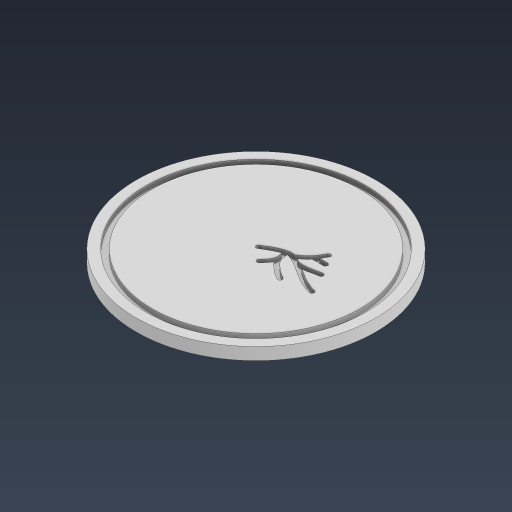
# Autodesk Inventor part: Podkladka_serce
Saved by Autodesk Inventor 2024 (Build 280153000, 153)
## iProperties
Created: 2023-12-26
Part Number: Podkladka_serce
Material: Generic
Document SubType Name: Modeling
Designer: Piter
Density: 1 g/cm^3
Appearance: Default
Author: Piter
Autodesk Inventor part; units mm, degrees
ref_plane "YZ Plane" through (0, 0, 0) normal (1, 0, 0) x (0, 1, 0)
ref_plane "XZ Plane" through (0, 0, 0) normal (0, 1, 0) x (-1, 0, 0)
ref_plane "XY Plane" through (0, 0, 0) normal (0, 0, 1) x (1, 0, 0)
sketch "Sketch1" plane through (0, 0, 0) normal (0, 1, 0) x (-1, 0, 0)
  circle A0 centre (0, 0) radius 49
  dimension "d0" = 98
  constraints: 1 centre point, 1 coincident
  measures "d0" diameter of A0
extrude "Extrusion1" add sketch "Sketch1" along normal blind 5
sketch "Sketch2" plane through (0, 5, 0) normal (0, 1, 0) x (1, 0, 0)
  circle A0 centre (0, 0) radius 45
  circle A1 centre (0, 0) radius 42.5
  dimension "d3" = 90
  dimension "d4" = 85
  constraints: 2 centre point, 2 coincident
  measures "d3" diameter of A0
  measures "d4" diameter of A1
extrude "Extrusion2" cut sketch "Sketch2" against normal blind 2
sketch "Sketch3" plane through (0, 5, 0) normal (0, 1, 0) x (1, 0, 0)
  line L0 (-57.9545, -56.5544) -> (-57.9545, 60.4671) construction
  line L1 (-57.9545, 60.4671) -> (59.0671, 60.4671) construction
  line L2 (59.0671, 60.4671) -> (59.0671, -56.5544) construction
  line L3 (59.0671, -56.5544) -> (-57.9545, -56.5544) construction
  spline S0 degree 4 poles (-30.855, -14.6939) (-30.5592, -15.2121) (-28.9514, -13.3397) (-26.9762, -13.2223) (-24.8329, -11.8951) (-22.2326, -11.9313) (-20.944, -12.0116) (-19.8559, -12.2221) (-18.785, -12.2474) (-17.611, -12.515) (-16.3643, -12.7351) (-15.334, -13.394) (-15.132, -13.7512) knots 0 0 0 0 0 0.211335 0.31885 0.420472 0.514533 0.599869 0.673378 0.744824 0.818641 1 1 1 1 1
  spline S1 degree 4 poles (-15.132, -13.7512) (-14.8227, -14.055) (-14.7175, -14.4119) (-14.2396, -15.0741) (-13.9799, -15.4717) (-13.6078, -15.8281) (-13.4414, -16.0861) (-13.1181, -16.4937) (-12.8312, -16.729) (-12.5324, -17.1008) (-12.243, -17.2913) (-11.898, -17.6305) (-11.433, -17.931) (-11.1614, -18.1872) (-10.7354, -18.4386) (-10.393, -18.6914) (-10.1007, -18.8902) (-9.6444, -19.1399) (-9.4269, -19.2823) (-8.8905, -19.4957) (-8.5475, -19.6618) (-8.2328, -19.8231) (-8.0583, -19.8821) knots 0 0 0 0 0 0.130277 0.178357 0.223468 0.267757 0.312685 0.357477 0.402319 0.447217 0.493758 0.540064 0.587831 0.634826 0.679831 0.725599 0.769028 0.811962 0.854881 0.896603 1 1 1 1 1
  spline S2 degree 4 poles (-8.0583, -19.8821) (-7.8236, -19.9246) (-7.3928, -20.2345) (-7.0213, -20.2224) (-6.4723, -20.5412) (-5.7818, -20.6348) (-4.0839, -21.2438) (-2.8883, -21.2479) (-2.0598, -21.5949) (3.0382, -21.8666) (4.3318, -21.5299) (5.1217, -21.4873) knots 0 0 0 0 0 0.143312 0.201694 0.275908 0.361306 0.452284 0.563274 0.684961 1 1 1 1 1
  spline S3 degree 4 poles (5.1217, -21.4873) (5.3502, -21.885) (7.9688, -22.2735) (9.7694, -21.9854) (13.5046, -20.8683) (15.0412, -20.3002) (18.2153, -18.4381) (18.9378, -17.9974) (21.8671, -15.9314) (23.6336, -14.3654) (24.9433, -13.2213) (28.1026, -10.9236) (30.8845, -9.4621) (34.5176, -7.4895) (35.0528, -6.595) (36.3359, -4.3458) knots 0 0 0 0 0 0.142124 0.208489 0.276802 0.341864 0.408085 0.475147 0.538695 0.609209 0.678841 0.750076 0.822266 1 1 1 1 1
  spline S4 degree 4 poles (36.3359, -4.3458) (36.7245, -3.6239) (36.8383, -0.8543) (35.4768, 2.2728) (32.0422, 7.8368) (27.8466, 12.0021) (23.4613, 16.0926) (18.9758, 17.9098) (17.0368, 19.1716) (10.9838, 20.2095) (4.2523, 20.1992) (2.4357, 19.9615) (-5.0655, 18.757) (-6.5918, 17.9988) knots 0 0 0 0 0 0.146469 0.225498 0.31307 0.401766 0.484157 0.564599 0.642138 0.717145 0.798076 1 1 1 1 1
  spline S5 degree 4 poles (-6.5918, 17.9988) (-6.4353, 18.6383) (-6.1547, 20.9102) (-5.4504, 22.2073) (-6.1351, 23.8716) (-6.9933, 24.7962) (-9.5292, 26.1955) (-12.2866, 25.8973) (-13.5339, 25.9509) (-14.161, 24.4612) knots 0 0 0 0 0 0.273717 0.372323 0.471117 0.581172 0.698617 1 1 1 1 1
  spline S6 degree 3 poles (-14.161, 24.4612) (-14.5628, 23.0574) (-14.5553, 22.1068) (-14.7653, 20.84) knots 0 0 0 0 1 1 1 1
  spline S7 degree 4 poles (-14.7653, 20.84) (-15.5966, 20.7471) (-17.1378, 20.7254) (-19.7431, 19.1266) (-21.6791, 17.0978) (-22.8834, 15.7469) (-23.5493, 14.46) (-23.8697, 14.0744) knots 0 0 0 0 0 0.373739 0.530619 0.681614 1 1 1 1 1
  spline S8 degree 2 poles (-23.8697, 14.0744) (-25.0153, 14.8562) (-26.0757, 15.4579) knots 0 0 0 1 1 1
  spline S9 degree 4 poles (-26.0757, 15.4579) (-26.3931, 15.5036) (-27.2913, 15.207) (-28.288, 15.2326) (-29.5466, 13.4746) (-29.3662, 13.1095) (-29.4752, 12.4274) knots 0 0 0 0 0 0.400545 0.573365 1 1 1 1 1
  spline S10 degree 4 poles (-29.4752, 12.4274) (-29.414, 11.9968) (-28.8884, 11.3655) (-28.1793, 10.512) (-26.8732, 9.0508) (-26.2826, 8.5073) (-25.8263, 7.7752) knots 0 0 0 0 0 0.376148 0.544005 1 1 1 1 1
  spline S11 degree 4 poles (-25.8263, 7.7752) (-25.8622, 6.8686) (-25.631, 5.5215) (-25.6166, 3.8587) (-25.165, 2.7629) (-25.0295, 2.1644) knots 0 0 0 0 0 0.526484 1 1 1 1 1
  spline S12 degree 4 poles (-25.0295, 2.1644) (-25.4773, 2.4387) (-26.3039, 3.4935) (-27.4328, 4.3276) (-28.4973, 5.9882) (-28.8964, 6.5508) (-29.2003, 6.5044) knots 0 0 0 0 0 0.456511 0.639346 1 1 1 1 1
  spline S13 degree 4 poles (-29.2003, 6.5044) (-29.2723, 6.6254) (-30.5043, 6.4492) (-30.6821, 6.5696) (-33.1305, 6.0924) (-34.1882, 5.4096) (-35.1291, 5.0929) (-35.6654, 4.3404) (-35.497, 3.2653) (-35.3332, 2.1398) (-34.847, 0.876) (-34.6637, 0.143) (-33.0685, -2.8394) (-32.1568, -3.4799) (-31.5129, -4.7983) (-30.855, -5.1324) knots 0 0 0 0 0 0.128955 0.197692 0.266621 0.335258 0.397687 0.4585 0.521575 0.586628 0.66007 0.736731 0.814417 1 1 1 1 1
  spline S14 degree 4 poles (-30.855, -5.1324) (-31.3072, -5.0811) (-32.4824, -6.0147) (-33.4416, -5.6132) (-34.4117, -6.5448) (-34.2011, -7.1991) (-34.5753, -7.9124) (-34.0851, -9.8836) (-33.8857, -10.6052) (-33.2722, -11.8795) (-33.1592, -12.1297) (-32.1294, -13.7542) (-31.5448, -14.1358) (-31.1758, -14.8275) (-30.855, -14.6939) knots 0 0 0 0 0 0.189822 0.256724 0.319063 0.3908 0.467513 0.549565 0.628853 0.703353 0.776714 0.846802 1 1 1 1 1
  spline S15 degree 4 poles (6.5616, 3.8895) (7.2445, 2.9756) (7.2461, 0.8391) (6.5311, -1.1769) (3.8219, -3.2437) (4.0337, -3.5283) knots 0 0 0 0 0 0.531588 1 1 1 1 1
  spline S16 degree 4 poles (4.0337, -3.5283) (4.0303, -3.7044) (3.977, -3.9973) (4.2401, -4.1161) (4.4241, -4.3894) (4.7928, -4.4957) (5.1648, -4.5306) (5.4925, -4.3648) (5.9212, -3.7895) (6.3103, -3.5675) (6.7668, -2.8806) (7.5526, -2.0547) (7.5449, -1.8316) (8.1211, -1.083) (8.1828, -0.8707) knots 0 0 0 0 0 0.135338 0.188896 0.24616 0.30712 0.376504 0.449718 0.531408 0.621269 0.707174 0.7946 1 1 1 1 1
  spline S17 degree 4 poles (8.1828, -0.8707) (8.4546, -1.208) (8.8667, -1.4974) (9.3887, -2.1927) (10.1496, -2.8061) (10.8622, -3.4963) (11.3704, -3.8355) (11.8724, -4.3064) (13.156, -5.3006) (13.8014, -5.6015) (14.59, -6.1647) (15.0515, -6.3971) knots 0 0 0 0 0 0.207696 0.297295 0.386448 0.47475 0.567307 0.659406 0.755636 1 1 1 1 1
  spline S18 degree 3 poles (15.0515, -6.3971) (15.4641, -6.5642) (15.5632, -6.3905) (15.9055, -6.2657) knots 0 0 0 0 1 1 1 1
  spline S19 degree 4 poles (15.9055, -6.2657) (16.2304, -6.266) (16.2383, -5.147) (16.3543, -5.0864) (15.3625, -4.4615) (15.2343, -4.4946) knots 0 0 0 0 0 0.502014 1 1 1 1 1
  spline S20 degree 4 poles (15.2343, -4.4946) (14.6789, -4.099) (13.7291, -3.5273) (12.1956, -2.3469) (11.3062, -1.4157) (9.6897, -0.0805) (9.4807, 0.5376) (8.799, 1.204) knots 0 0 0 0 0 0.361166 0.503734 0.642443 1 1 1 1 1
  spline S21 degree 4 poles (8.799, 1.204) (8.9618, 1.5458) (8.7409, 2.4091) (8.8564, 3.0664) (8.4394, 3.8869) (8.4004, 4.1762) knots 0 0 0 0 0 0.506238 1 1 1 1 1
  spline S22 degree 4 poles (8.4004, 4.1762) (8.5385, 4.378) (8.8982, 4.0785) (9.3675, 4.2651) (10.0273, 3.8367) (11.2034, 3.4779) (11.3206, 3.1849) (13.3538, 2.3413) (14.5675, 1.3511) (16.0887, 0.4784) (17.5876, -0.4575) (19.4986, -1.6168) (21.4732, -2.9511) (22.7081, -3.1766) (23.9472, -3.7779) knots 0 0 0 0 0 0.09874 0.149623 0.202515 0.266535 0.340903 0.420474 0.509585 0.598304 0.68637 0.774222 1 1 1 1 1
  spline S23 degree 4 poles (23.9472, -3.7779) (24.2439, -4.0577) (25.1334, -4.1522) (25.333, -4.398) (26.4858, -4.5531) (26.9248, -4.5649) (27.2302, -4.2956) (27.5476, -3.9393) (27.4526, -3.4628) (27.4189, -3.2229) (27.0176, -2.7705) (26.8652, -2.8422) (26.3055, -2.6913) (26.1129, -2.7091) knots 0 0 0 0 0 0.234782 0.321807 0.40375 0.484284 0.558275 0.628906 0.698735 0.762766 0.825285 1 1 1 1 1
  spline S24 degree 4 poles (26.1129, -2.7091) (25.9385, -2.7567) (24.9702, -2.2913) (24.6698, -2.1739) (23.0465, -1.4361) (22.0932, -1.164) (21.0175, -0.4574) (20.1997, -0.2185) (19.0929, 0.7946) (18.793, 0.7294) (17.7456, 1.5293) (17.6493, 1.5365) (16.4566, 2.3576) (16.4847, 2.2841) knots 0 0 0 0 0 0.174457 0.258499 0.346709 0.439959 0.532461 0.615733 0.693831 0.764781 0.834294 1 1 1 1 1
  spline S25 degree 4 poles (16.4847, 2.2841) (17.0349, 2.4087) (17.9121, 2.318) (18.9957, 2.6619) (21.158, 3.0971) (22.5194, 3.3919) (22.6843, 3.3009) knots 0 0 0 0 0 0.400135 0.583018 1 1 1 1 1
  spline S26 degree 4 poles (22.6843, 3.3009) (22.9805, 3.4989) (23.0187, 3.2696) (23.7927, 4.6642) (22.7582, 4.9379) (22.7566, 5.1138) (22.3847, 5.0756) knots 0 0 0 0 0 0.41069 0.585007 1 1 1 1 1
  circle A0 centre (19.663, 8.7711) radius 0.912
  circle A1 centre (17.1461, 12.6093) radius 0.8322
  line L4 (16.4209, 9.6831) -> (19.663, 9.6831)
  line L5 (16.4209, 9.6831) -> (17.8672, 12.1939)
  line L6 (15.1581, 7.8591) -> (19.663, 7.8591)
  spline S27 degree 4 poles (22.3847, 5.0756) (21.9386, 5.0986) (19.7162, 4.5168) (18.9321, 4.5221) (17.1645, 4.0519) (15.6452, 4.1276) (14.6647, 3.8742) (13.8321, 4.1524) (13.4679, 4.107) knots 0 0 0 0 0 0.350728 0.484058 0.608102 0.730562 1 1 1 1 1
  spline S28 degree 2 poles (13.4679, 4.107) (12.6648, 4.6192) (11.8619, 5.0249) knots 0 0 0 1 1 1
  spline S29 degree 2 poles (11.8619, 5.0249) (13.5779, 5.9848) (15.1581, 7.8591) knots 0 0 0 1 1 1
  spline S30 degree 4 poles (16.425, 13.0246) (15.7809, 12.0877) (14.636, 9.3288) (12.462, 7.7178) (10.8241, 6.3091) (9.7155, 5.8429) knots 0 0 0 0 0 0.51347 1 1 1 1 1
  spline S31 degree 4 poles (9.7155, 5.8429) (8.7697, 6.2661) (5.9257, 5.602) (3.0817, 4.6798) (0.1827, 2.396) (-0.9318, 1.8757) knots 0 0 0 0 0 0.474829 1 1 1 1 1
  circle A2 centre (-0.2991, 1.254) radius 0.8879
  spline S32 degree 2 poles (0.0834, 0.4527) (3.5128, 2.5638) (6.5616, 3.8895) knots 0 0 0 1 1 1
  spline S33 degree 4 poles (2.9679, -19.7591) (2.2419, -17.8923) (0.9961, -12.1009) (-7.2544, -10.462) (-16.8725, -7.6679) (-22.0178, -5.2731) (-23.8697, -0.5291) knots 0 0 0 0 0 0.378657 0.547911 1 1 1 1 1
  spline S34 degree 4 poles (-23.8697, -0.5291) (-26.1643, -0.0299) (-27.382, 2.3303) (-29.339, 3.663) (-29.8326, 4.8452) knots 0 0 0 0 0 1 1 1 1 1
  spline S35 degree 3 poles (-29.8326, 4.8452) (-31.1171, 4.6647) (-32.8029, 4.6123) (-33.7457, 3.6682) knots 0 0 0 0 1 1 1 1
  spline S36 degree 4 poles (-33.7457, 3.6682) (-33.9956, 2.9658) (-33.0323, 1.3268) (-32.4613, -1.0963) (-30.5129, -2.4971) (-30.2427, -3.87) (-29.0662, -4.5411) knots 0 0 0 0 0 0.412269 0.579381 1 1 1 1 1
  spline S37 degree 4 poles (-29.0662, -4.5411) (-28.5415, -4.5867) (-27.5718, -4.0236) (-27.1921, -4.1231) (-26.5877, -3.8956) knots 0 0 0 0 0 1 1 1 1 1
  spline S38 degree 4 poles (-26.5877, -3.8956) (-26.3846, -3.8438) (-25.8545, -3.8821) (-25.7283, -4.1535) (-25.3514, -4.7592) (-25.5834, -5.4102) (-25.8656, -5.4159) (-25.9944, -5.597) knots 0 0 0 0 0 0.360536 0.505378 0.649978 1 1 1 1 1
  spline S39 degree 4 poles (-25.9944, -5.597) (-26.2135, -5.6619) (-29.9686, -6.6351) (-28.688, -6.3543) (-32.4517, -7.5419) (-32.5612, -7.5505) knots 0 0 0 0 0 0.506465 1 1 1 1 1
  spline S40 degree 4 poles (-32.5612, -7.5505) (-32.5942, -8.2713) (-32.4836, -9.0562) (-32.1777, -10.1767) (-31.4756, -11.3772) (-31.1628, -12.1302) (-30.6329, -12.5387) (-30.556, -12.7403) knots 0 0 0 0 0 0.401034 0.550759 0.694254 1 1 1 1 1
  spline S41 degree 4 poles (-30.556, -12.7403) (-30.1826, -12.6443) (-29.5482, -11.9983) (-28.8304, -11.8666) (-27.9715, -11.3926) (-27.1896, -11.0818) (-26.3609, -10.7012) (-25.3281, -10.4749) (-23.18, -10.0528) (-22.1628, -10.2876) (-20.3428, -10.2474) (-18.6193, -10.4761) (-17.0267, -10.7801) (-15.2073, -11.3604) (-14.2323, -12.1196) (-13.0966, -13.2061) (-12.8974, -14.3013) (-11.3334, -15.7174) (-10.3073, -16.4994) (-8.988, -17.6871) (-6.3002, -18.7119) (-1.9787, -20.0364) (0.1251, -19.6586) (1.5341, -20.2075) (2.9679, -19.7591) knots 0 0 0 0 0 0.07385 0.1032 0.132674 0.164383 0.201354 0.240465 0.28268 0.327257 0.370931 0.416362 0.460647 0.503267 0.54381 0.584499 0.625417 0.667176 0.714377 0.766583 0.821627 0.876885 1 1 1 1 1
  spline S42 degree 4 poles (2.2296, -13.8729) (0.45, -10.5125) (-3.3187, -8.5558) (-8.1307, -8.8141) (-14.3146, -6.3967) knots 0 0 0 0 0 1 1 1 1 1
  spline S43 degree 4 poles (-14.3146, -6.3967) (-17.5338, -5.4136) (-19.9084, -3.4763) (-22.0027, -1.3922) (-24.6826, 5.8201) (-23.0718, 10.0392) (-26.306, 9.6652) (-27.6724, 12.6093) knots 0 0 0 0 0 0.376526 0.519789 0.656405 1 1 1 1 1
  spline S44 degree 2 poles (-27.6724, 12.6093) (-27.4326, 13.4428) (-26.4391, 13.6355) knots 0 0 0 1 1 1
  spline S45 degree 3 poles (-26.4391, 13.6355) (-25.7595, 13.2919) (-23.5767, 11.0928) (-22.4751, 12.8258) knots 0 0 0 0 1 1 1 1
  spline S46 degree 3 poles (-22.4751, 12.8258) (-21.2788, 15.2793) (-18.0738, 18.8143) (-15.132, 18.9717) knots 0 0 0 0 1 1 1 1
  line L7 (-15.132, 18.9717) -> (-16.7238, 7.8641)
  spline S47 degree 4 poles (-16.7238, 7.8641) (-17.0381, 6.4422) (-16.4824, 2.308) (-13.2012, -1.7139) (-9.6509, -2.7861) (-7.4047, -3.6311) knots 0 0 0 0 0 0.480437 1 1 1 1 1
  circle A3 centre (-7.4047, -2.7647) radius 0.9157
  spline S48 degree 4 poles (-7.4047, -1.849) (-8.5722, -1.3576) (-11.6797, -0.5151) (-14.1348, 3.0449) (-15.3959, 5.8416) (-14.9257, 9.9328) (-14.463, 11.1641) knots 0 0 0 0 0 0.408713 0.573926 1 1 1 1 1
  line L8 (-14.463, 11.1641) -> (-13.0046, 21.3408)
  spline S49 degree 3 poles (-13.0046, 21.3408) (-11.7938, 20.323) (-9.2226, 20.1747) (-7.9306, 20.3476) knots 0 0 0 0 1 1 1 1
  spline S50 degree 5 poles (-12.428, 24.0077) (-12.6133, 23.7848) (-12.5965, 23.2666) (-11.7794, 22.3001) (-11.0846, 22.481) (-7.6968, 21.6442) (-7.0077, 22.9263) (-8.7203, 23.9413) (-11.3044, 24.5181) (-12.1943, 24.2889) (-12.428, 24.0077) knots 0 0 0 0 0 0 0.179978 0.299331 0.454344 0.62904 0.77301 1 1 1 1 1 1
  spline S51 degree 4 poles (-7.9306, 20.3476) (-7.8562, 19.2448) (-9.2277, 12.9247) (-7.1671, 8.845) (-5.4315, 5.6453) (-0.0385, 6.7984) (1.3531, 6.7251) knots 0 0 0 0 0 0.439272 0.598207 1 1 1 1 1
  circle A4 centre (1.0311, 7.6121) radius 0.9502
  spline S52 degree 4 poles (0.5888, 8.4531) (-2.9906, 8.9735) (-5.8493, 5.6123) (-7.0367, 12.3908) (-6.489, 16.1151) knots 0 0 0 0 0 1 1 1 1 1
  spline S53 degree 4 poles (-6.489, 16.1151) (-4.0176, 16.7764) (0.3382, 18.3948) (6.7153, 18.3794) (11.1448, 18.414) (14.0627, 17.6728) (17.9608, 17.0911) (21.9035, 14.4082) (28.0542, 10.3268) (30.6729, 5.8017) (34.221, 1.973) (34.7495, -1.7716) knots 0 0 0 0 0 0.233698 0.318044 0.396968 0.476435 0.562637 0.65479 0.751021 1 1 1 1 1
  spline S54 degree 4 poles (34.7495, -1.7716) (34.7834, -4.6398) (34.317, -5.5808) (25.8366, -10.1311) (22.9115, -12.6009) (20.0293, -15.2767) (16.4894, -17.2928) (14.0062, -18.9692) (10.1177, -20.0229) (7.9441, -20.7915) (5.3276, -19.9482) (4.7584, -19.1358) knots 0 0 0 0 0 0.249724 0.354426 0.459159 0.553257 0.645725 0.73357 0.815578 1 1 1 1 1
  spline S55 degree 4 poles (4.7584, -19.1358) (4.538, -18.9616) (4.0062, -17.8841) (3.7117, -16.9683) (3.5683, -16.1566) (3.321, -15.8818) knots 0 0 0 0 0 0.511666 1 1 1 1 1
  point P0 (0, 0)
  point P1 (-30.3089, -14.6938)
  point P2 (-28.4652, -13.5676)
  point P3 (-26.5873, -12.817)
  point P4 (-24.573, -12.1005)
  point P5 (-22.0684, -11.9571)
  point P6 (-20.7633, -12.0659)
  point P7 (-19.7628, -12.1963)
  point P8 (-18.8058, -12.2833)
  point P9 (-17.9524, -12.4319)
  point P10 (-16.9207, -12.6829)
  point P11 (-15.7425, -13.2063)
  point P12 (-14.7653, -14.2432)
  point P13 (-14.4631, -14.7491)
  point P14 (-14.161, -15.1988)
  point P15 (-13.9361, -15.494)
  point P16 (-13.641, -15.8172)
  point P17 (-13.4232, -16.0983)
  point P18 (-13.1211, -16.4637)
  point P19 (-12.8259, -16.7588)
  point P20 (-12.5308, -17.0679)
  point P21 (-12.2568, -17.2998)
  point P22 (-11.8914, -17.609)
  point P23 (-11.4515, -17.9373)
  point P24 (-11.1276, -18.1883)
  point P25 (-10.7389, -18.4475)
  point P26 (-10.3947, -18.6863)
  point P27 (-10.0668, -18.9009)
  point P28 (-9.6619, -19.1358)
  point P29 (-9.3987, -19.2816)
  point P30 (-9.0485, -19.4362)
  point P31 (-8.6918, -19.5961)
  point P32 (-8.3504, -19.7591)
  point P33 (-7.6168, -20.0615)
  point P34 (-7.223, -20.2229)
  point P35 (-6.9287, -20.3138)
  point P36 (-6.5929, -20.4503)
  point P37 (-5.9624, -20.6326)
  point P38 (-4.1721, -21.1264)
  point P39 (-3.0669, -21.2878)
  point P40 (-2.3502, -21.4072)
  point P41 (0.5557, -21.6678)
  point P42 (3.9507, -21.6025)
  point P43 (6.0165, -21.8763)
  point P44 (8.3729, -22.0515)
  point P45 (10.6904, -21.6687)
  point P46 (13.2999, -20.9025)
  point P47 (15.3253, -20.0618)
  point P48 (17.9027, -18.6152)
  point P49 (19.1784, -17.8075)
  point P50 (21.6801, -15.996)
  point P51 (23.551, -14.4424)
  point P52 (25.0389, -13.2057)
  point P53 (27.911, -11.1495)
  point P54 (30.3383, -9.7412)
  point P55 (32.8769, -8.2959)
  point P56 (34.6001, -6.9433)
  point P57 (36.6183, -3.0278)
  point P58 (36.3359, -0.4544)
  point P59 (35.0178, 2.778)
  point P60 (32.162, 7.2344)
  point P61 (27.6114, 12.1616)
  point P62 (22.6843, 16.1158)
  point P63 (19.1785, 17.936)
  point P64 (16.7215, 18.9717)
  point P65 (11.1354, 20.0073)
  point P66 (6.271, 20.1642)
  point P67 (3.321, 19.9759)
  point P68 (-1.7317, 19.2228)
  point P69 (-6.2629, 19.7278)
  point P70 (-5.8612, 21.6665)
  point P71 (-5.8, 22.7668)
  point P72 (-6.1493, 23.7186)
  point P73 (-6.9278, 24.6095)
  point P74 (-8.6917, 25.5615)
  point P75 (-11.1276, 25.9284)
  point P76 (-12.9338, 25.728)
  point P77 (-14.463, 23.0985)
  point P78 (-14.6068, 22.0111)
  point P79 (-16.0684, 20.6746)
  point P80 (-18.0802, 19.975)
  point P81 (-20.145, 18.5915)
  point P82 (-21.4158, 17.3562)
  point P83 (-22.4749, 16.1151)
  point P84 (-23.3576, 14.8329)
  point P85 (-25.0295, 14.8334)
  point P86 (-26.6882, 15.3923)
  point P87 (-27.5278, 15.184)
  point P88 (-28.2783, 14.8326)
  point P89 (-29.066, 13.9948)
  point P90 (-29.3783, 13.2593)
  point P91 (-29.2003, 11.7958)
  point P92 (-28.7172, 11.1641)
  point P93 (-28.1599, 10.5101)
  point P94 (-27.387, 9.6406)
  point P95 (-26.5878, 8.7711)
  point P96 (-25.7742, 6.3854)
  point P97 (-25.6478, 5.1665)
  point P98 (-25.4917, 4.0072)
  point P99 (-25.2689, 3.0412)
  point P100 (-25.7743, 2.8332)
  point P101 (-26.6884, 3.7771)
  point P102 (-27.5282, 4.669)
  point P103 (-28.3309, 5.7318)
  point P104 (-28.8734, 6.3857)
  point P105 (-29.5347, 6.5564)
  point P106 (-30.3893, 6.5044)
  point P107 (-31.1548, 6.4375)
  point P108 (-33.0294, 6)
  point P109 (-34.3469, 5.3912)
  point P110 (-35.1101, 4.9551)
  point P111 (-35.5099, 4.3372)
  point P112 (-35.5099, 3.3558)
  point P113 (-35.2827, 2.1643)
  point P114 (-34.9283, 1.0479)
  point P115 (-34.5921, 0.1393)
  point P116 (-33.4843, -1.912)
  point P117 (-32.4771, -3.2922)
  point P118 (-31.686, -4.3459)
  point P119 (-31.8632, -5.4659)
  point P120 (-33.0294, -5.8333)
  point P121 (-33.7982, -6.0628)
  point P122 (-34.2442, -6.5613)
  point P123 (-34.3033, -7.0795)
  point P124 (-34.3951, -7.8207)
  point P125 (-34.113, -9.7413)
  point P126 (-33.7457, -10.8512)
  point P127 (-33.3259, -11.7695)
  point P128 (-33.0847, -12.2249)
  point P129 (-32.3617, -13.3044)
  point P130 (-31.6861, -14.098)
  point P131 (-31.2138, -14.6031)
  point P132 (7.0987, 2.3754)
  point P133 (6.887, 0.6816)
  point P134 (5.8774, -1.2242)
  point P135 (4.2654, -3.028)
  point P136 (4.0337, -3.8434)
  point P137 (4.1177, -4.0429)
  point P138 (4.2652, -4.1899)
  point P139 (4.4328, -4.3458)
  point P140 (4.7584, -4.4735)
  point P141 (5.1216, -4.4945)
  point P142 (5.4412, -4.3457)
  point P143 (5.8775, -3.8958)
  point P144 (6.2709, -3.5282)
  point P145 (6.8067, -2.8769)
  point P146 (7.3214, -2.2572)
  point P147 (7.5525, -1.9119)
  point P148 (7.8887, -1.3854)
  point P149 (8.6148, -1.3227)
  point P150 (9.0636, -1.7716)
  point P151 (9.5679, -2.298)
  point P152 (10.1663, -2.841)
  point P153 (10.87, -3.4671)
  point P154 (11.3465, -3.8434)
  point P155 (11.8619, -4.2761)
  point P156 (12.7616, -4.9706)
  point P157 (13.5218, -5.4659)
  point P158 (14.2726, -5.9372)
  point P159 (15.408, -6.4625)
  point P160 (15.6144, -6.3967)
  point P161 (16.1878, -5.9373)
  point P162 (16.2165, -5.354)
  point P163 (16.0793, -5.0218)
  point P164 (15.6145, -4.6461)
  point P165 (14.2726, -3.8434)
  point P166 (13.0097, -2.9417)
  point P167 (12.0419, -2.1472)
  point P168 (11.4425, -1.5911)
  point P169 (10.4747, -0.6955)
  point P170 (9.6224, 0.2434)
  point P171 (8.8767, 1.7984)
  point P172 (8.8101, 2.4435)
  point P173 (8.7217, 3.0479)
  point P174 (8.5467, 3.6685)
  point P175 (8.6422, 4.2557)
  point P176 (9.0142, 4.1762)
  point P177 (9.4187, 4.1257)
  point P178 (9.9965, 3.9005)
  point P179 (10.9499, 3.5117)
  point P180 (11.4193, 3.2373)
  point P181 (12.9357, 2.45)
  point P182 (14.6125, 1.3859)
  point P183 (16.1068, 0.4527)
  point P184 (17.5725, -0.4434)
  point P185 (18.9723, -1.3118)
  point P186 (20.5762, -2.287)
  point P187 (22.137, -3.0278)
  point P188 (24.6528, -4.0977)
  point P189 (25.2461, -4.2755)
  point P190 (25.7393, -4.4261)
  point P191 (26.5114, -4.5402)
  point P192 (26.9331, -4.4933)
  point P193 (27.2335, -4.2749)
  point P194 (27.4695, -3.8947)
  point P195 (27.4553, -3.4662)
  point P196 (27.3625, -3.1964)
  point P197 (27.1409, -2.9412)
  point P198 (26.948, -2.8406)
  point P199 (26.5937, -2.7646)
  constraints: 10 end point, 4 point on circle, 2 centre point, 2 tangent, 1 parallel, 1 vertical alignment, 479 other
extrude "Extrusion3" cut sketch "Sketch3" against normal blind 2 contours S32 A2 S31 S30 A1 L5 L4 A0 L6 S29 S28 S27 S26 S25 S24 S23 S22 S21 S20 S19 S18 S17 S16 S15 | S32 A2 S31 | A2 S31 | A1 | A0
body "Solid1"
